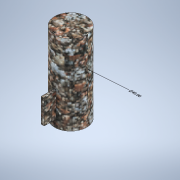
# Autodesk Inventor part: fuel
Saved by Autodesk Inventor 2022 (Build 260153000, 153)
## iProperties
Created: 2021-09-20
Part Number: fuel
Material: PAEK Plastic
Document SubType Name: Modeling
Designer: WASHINGTON
Density: 1.32 g/cm^3
Appearance: With Stone 1
Author: WASHINGTON
Autodesk Inventor part; units mm, degrees
ref_plane "YZ Plane" through (0, 0, 0) normal (1, 0, 0) x (0, 1, 0)
ref_plane "XZ Plane" through (0, 0, 0) normal (0, 1, 0) x (-1, 0, 0)
sketch "Sketch1" plane through (0, 0, 0) normal (0, 1, 0) x (-1, 0, 0)
  circle A0 centre (0, 0) radius 20
  dimension "d0" = 40
  constraints: 1 centre point, 1 coincident
  measures "d0" diameter of A0
extrude "Extrusion1" add sketch "Sketch1" along normal mid plane 100
ref_plane "Work Plane1" through (0, 0, 20) normal (0, 0, 1) x (1, 0, 0)
sketch "Sketch2" plane through (0, 0, 20) normal (0, 0, 1) x (1, 0, 0)
  line L0 (-2, -10) -> (2, -10)
  line L1 (2, -10) -> (2, -40)
  line L2 (2, -40) -> (-2, -40)
  line L3 (-2, -40) -> (-2, -10)
  point P0 (0, 0)
  dimension "d3" = 4
  dimension "d4" = 2
  dimension "d5" = 30
  dimension "d6" = 10
  constraints: 8 end point, 2 parallel, 1 horizontal, 1 perpendicular
  measures "d3" distance of L0.start L0.end
  measures "d4" distance from line of point (0, 0) L1
  measures "d5" distance of L0.end L1.end
  measures "d6" distance from line of point (0, 0) L0
extrude "Extrusion2" add sketch "Sketch2" along normal blind 15 and the other way blind 5
body "Solid1"
